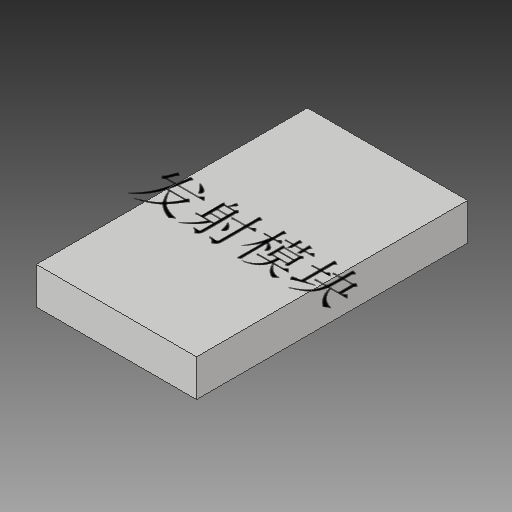
# Autodesk Inventor part: 无线发射模块
Saved by Autodesk Inventor 2018 (Build 220112000, 112)
## iProperties
Created: 2020-11-25
Part Number: 无线发射模块
Material: 常规
Document SubType Name: Modeling
Designer: OHHHHHHHHHH
Density: 1 g/cm^3
Appearance: 默认
Author: OHHHHHHHHHH
Autodesk Inventor part; units mm, degrees
ref_plane "YZ Plane" through (0, 0, 0) normal (1, 0, 0) x (0, 1, 0)
ref_plane "XZ Plane" through (0, 0, 0) normal (0, 1, 0) x (-1, 0, 0)
ref_plane "XY Plane" through (0, 0, 0) normal (0, 0, 1) x (1, 0, 0)
sketch "草图1" plane through (0, 0, 0) normal (0, 1, 0) x (-1, 0, 0)
  line L0 (0, 0) -> (13, 0)
  line L1 (13, 0) -> (13, -22)
  line L2 (13, -22) -> (0, -22)
  line L3 (0, -22) -> (0, 0)
  dimension "d0" = 22
  dimension "d1" = 13
  constraints: 8 end point, 2 parallel, 1 horizontal, 1 perpendicular
  measures "d0" distance of L0.end L1.end
  measures "d1" distance of L0.start L0.end
extrude "拉伸1" add sketch "草图1" along normal blind 3
sketch "草图2" plane through (0, 3, 0) normal (0, 1, 0) x (1, 0, 0)
  line L0 (-14.56, 12.451) -> (2.2065, 12.451) construction
  line L1 (2.2065, 12.451) -> (2.2065, 8.5706) construction
  line L2 (2.2065, 8.5706) -> (-14.56, 8.5706) construction
  line L3 (-14.56, 8.5706) -> (-14.56, 12.451) construction
  constraints: 2 other
